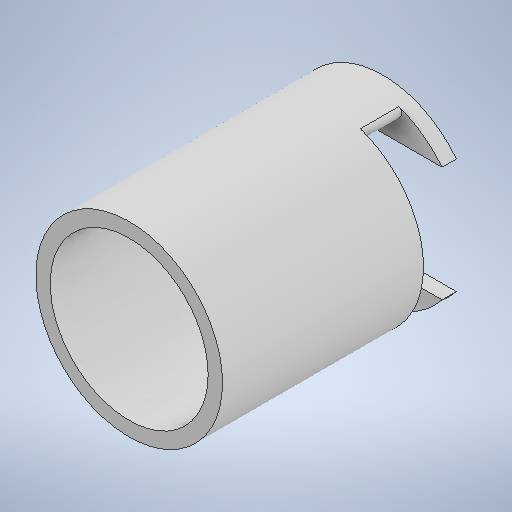
# Autodesk Inventor part: Tube_Test
Saved by Autodesk Inventor 2025.1 (Build 291241020, 241B)
## iProperties
Created: 2024-11-22
Part Number: Tube_Test
Material: Generic
Document SubType Name: Modeling
Designer: leon-
Density: 1 g/cm^3
Appearance: Default
Author: leon-
Autodesk Inventor part; units mm, degrees
ref_plane "YZ Plane" through (0, 0, 0) normal (1, 0, 0) x (0, 1, 0)
ref_plane "XZ Plane" through (0, 0, 0) normal (0, 1, 0) x (-1, 0, 0)
ref_plane "XY Plane" through (0, 0, 0) normal (0, 0, 1) x (1, 0, 0)
sketch "Sketch1" plane through (0, 0, 0) normal (0, 0, 1) x (1, 0, 0)
  circle A0 centre (0, 0) radius 16.5
  circle A1 centre (0, 0) radius 19.5
  dimension "d0" = 33
  dimension "d1" = 39
  constraints: 2 centre point, 2 coincident
  measures "d0" diameter of A0
  measures "d1" diameter of A1
extrude "Extrusion1" add sketch "Sketch1" along normal blind 50
sketch "Sketch2" plane through (0, 0, 0) normal (0, 0, -1) x (-1, 0, 0)
  circle A0 centre (0, 0) radius 19.5
  constraints: 1 centre point, 1 coincident
extrude "Extrusion2" add sketch "Sketch2" along normal blind 3
sketch "Sketch3" plane through (0, 0, 0) normal (1, 0, 0) x (0, 1, 0)
  line L0 (-16.5, 0) -> (16.5, 0) projected
  line L1 (16.5, 0) -> (-16.5, 0)
  line L2 (-16.5, 0) -> (-16.5, 8)
  line L3 (-16.5, 8) -> (16.5, 8)
  line L4 (16.5, 8) -> (16.5, 0)
  point P0 (0, 0)
  dimension "d6" = 8
  constraints: 8 end point, 2 parallel, 1 horizontal, 1 perpendicular
  measures "d6" distance between parallel lines of L0 L3
extrude "Extrusion3" cut sketch "Sketch3" along normal through all
sketch "Sketch4" plane through (0, 0, -3) normal (0, 0, -1) x (-1, 0, 0)
  circle A0 centre (0, 0) radius 12
  line L0 (0, 12) -> (-19.5, 12)
  line L1 (-19.5, 12) -> (-19.5, -12)
  line L2 (-19.5, -12) -> (0, -12)
  point P0 (-19.5, 0)
  dimension "d9" = 24
  dimension "d10" = 19.5
  constraints: 6 end point, 2 horizontal, 2 point on circle, 2 tangent, 1 centre point, 1 coincident, 1 midpoint, 1 perpendicular
  measures "d9" diameter of A0
  measures "d10" distance of point (0, 0) point (-19.5, 0)
extrude "Extrusion4" cut sketch "Sketch4" against normal blind 10
fillet "Fillet1" radius 1 2 edges at (10.3923, -16.5, 4) (10.3923, 16.5, 4)
fillet "Fillet2" radius 1 2 edges at (11.6673, 11.6673, 8) (11.6673, -11.6673, 8)
body "Solid1"
